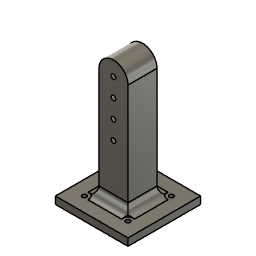
camera stand v4 (Autodesk Fusion 360 design; units mm, degrees)
Autodesk Fusion 360 part; units mm, degrees
sketch "Sketch1" plane through (0, 0, 0) normal (0, 1, 0) x (1, 0, 0)
  line L0 (0, 0) -> (50, 0)
  line L1 (50, 0) -> (50, -50)
  line L2 (50, -50) -> (0, -50)
  line L3 (0, -50) -> (0, 0)
  dimension "d1" = 50
  dimension "d2" = 50
  constraint horizontal L0
  constraint vertical L1
  constraint horizontal L2
  constraint vertical L3
  constraint coincident L0.start L3.end
  measures "d1" distance of L0.start L0.end
  measures "d2" distance of L0.start L2.end
extrude "Extrude1" add sketch "Sketch1" along normal blind 5
sketch "Sketch2" plane through (0, 5, 0) normal (0, 1, 0) x (-1, 0, 0)
  line L0 (0, 50) -> (-50, 50)
  line L1 (-50, 50) -> (-50, 0)
  line L2 (-50, 0) -> (0, 0)
  line L3 (0, 0) -> (0, 50)
  line L4 (-35.0043, 15.0162) -> (-15.0043, 15.0162)
  line L5 (-15.0043, 15.0162) -> (-15.0043, 35.0162)
  line L6 (-15.0043, 35.0162) -> (-35.0043, 35.0162)
  line L7 (-35.0043, 35.0162) -> (-35.0043, 15.0162)
  line L8 (-35.0043, 15.0162) -> (-15.0043, 35.0162) construction
  line L9 (-15.0043, 15.0162) -> (-35.0043, 35.0162) construction
  point P0 (-25.0043, 25.0162)
  dimension "d5" = 20
  dimension "d6" = 20
  constraint horizontal L4
  constraint perpendicular L4 L5
  constraint parallel L4 L6
  constraint parallel L5 L7
  constraint coincident L8 P0
  constraint coincident L9 P0
  measures "d5" distance of L5.end L6.end
  measures "d6" distance of L4.end L5.end
extrude "Extrude2" add sketch "Sketch2" along normal blind 76.2 contours L4 L5 L6 L7
sketch "Sketch3" plane through (0, 0, 35.0162) normal (0, 0, 1) x (1, 0, 0)
  line L0 (15.0043, 5) -> (35.0043, 5)
  line L1 (35.0043, 5) -> (35.0043, 81.2)
  line L2 (35.0043, 81.2) -> (15.0043, 81.2)
  line L3 (15.0043, 81.2) -> (15.0043, 5)
  arc A0 (35.0043, 81.2) -> (15.0043, 81.2) centre (25.0043, 81.2) ccw
  constraint midpoint L2 A0.centre
extrude "Extrude3" add sketch "Sketch3" against normal blind 20 contours L2 A0
sketch "Sketch4" plane through (0, 0, 35.0162) normal (0, 0, 1) x (1, 0, 0)
  line L0 (15.0043, 5) -> (35.0043, 5)
  line L1 (35.0043, 5) -> (35.0043, 81.2)
  arc A0 (35.0043, 81.2) -> (15.0043, 81.2) centre (25.0043, 81.2) ccw
  line L2 (15.0043, 81.2) -> (15.0043, 5)
  circle A1 centre (25.0043, 81.2) radius 1.6
  dimension "d11" = 3.2
  constraint concentric A0 A1
  measures "d11" diameter of A1
extrude "Extrude4" cut sketch "Sketch4" against normal blind 70 contours A1
pattern_linear "R-Pattern1" count 4 spacing 12.7 along (0, -1, 0) of "Extrude4"
sketch "Sketch5" plane through (0, 0, 0) normal (0, -1, 0) x (1, 0, 0)
  line L0 (50, 50) -> (0, 50)
  line L1 (0, 50) -> (0, 0)
  line L2 (0, 0) -> (50, 0)
  line L3 (50, 0) -> (50, 50)
  circle A0 centre (10, 10) radius 1.5
  circle A1 centre (10, 40) radius 1.5
  circle A2 centre (40, 10) radius 1.5
  circle A3 centre (40, 40) radius 1.5
  line L4 (10, 40) -> (40, 40)
  dimension "d18" = 3
  dimension "d20" = 3
  dimension "d21" = 30
  dimension "d22" = 3
  dimension "d23" = 3
  dimension "d24" = 30
  dimension "d25" = 30
  dimension "d26" = 30
  constraint coincident A1.centre L4.start
  constraint coincident A3.centre L4.end
  measures "d18" diameter of A0
  measures "d20" diameter of A1
  measures "d21" distance of A0.centre A1.centre
  measures "d22" diameter of A2
  measures "d23" diameter of A3
  measures "d24" distance of A2.centre A3.centre
  measures "d25" distance of A0.centre A2.centre
  measures "d26" horizontal distance of A1.centre A3.centre
extrude "Extrude5" cut sketch "Sketch5" against normal blind 25 contours A0 | A1 | A2 | A3
sketch "Sketch6" plane through (0, 5, 0) normal (0, 1, 0) x (-1, 0, 0)
  circle A0 centre (-10, 10) radius 1.5
  circle A1 centre (-10, 40) radius 1.5
  circle A2 centre (-40, 10) radius 1.5
  circle A3 centre (-40, 40) radius 1.5
  line L0 (-35.0043, 35.0162) -> (-15.0043, 35.0162)
  line L1 (-15.0043, 35.0162) -> (-15.0043, 15.0162)
  line L2 (-15.0043, 15.0162) -> (-35.0043, 15.0162)
  line L3 (-35.0043, 15.0162) -> (-35.0043, 35.0162)
  line L4 (0, 50) -> (-50, 50)
  line L5 (-50, 50) -> (-50, 0)
  line L6 (-50, 0) -> (0, 0)
  line L7 (0, 0) -> (0, 50)
  circle A4 centre (-10, 40) radius 3.5
  circle A5 centre (-40, 40) radius 3.5
  circle A6 centre (-40, 10) radius 3.5
  circle A7 centre (-10, 10) radius 3.5
  dimension "d31" = 7
  dimension "d32" = 7
  dimension "d33" = 7
  dimension "d34" = 7
  constraint concentric A1 A4
  constraint concentric A3 A5
  constraint concentric A2 A6
  constraint concentric A0 A7
  measures "d31" diameter of A4
  measures "d32" diameter of A5
  measures "d33" diameter of A6
  measures "d34" diameter of A7
fillet "Fillet1" radius 6 4 edges at (25.0043, 5, 35.0162) (35.0043, 5, 25.0162) (15.0043, 5, 25.0162) (25.0043, 5, 15.0162)
extrude "Extrude6" cut sketch "Sketch6" along normal blind 5 contours A4 | A5 | A6 | A7
